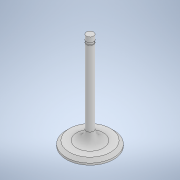
# Autodesk Inventor part: выпускной_клапан
Saved by Autodesk Inventor 2021 (Build 250183000, 183)
## iProperties
Created: 2020-12-20
Part Number: выпускной_клапан
Material: Типовые
Document SubType Name: Modeling
Designer: panda
Density: 1 g/cm^3
Appearance: По умолчанию
Author: panda
Autodesk Inventor part; units mm, degrees
ref_plane "YZ Plane" through (0, 0, 0) normal (1, 0, 0) x (0, 1, 0)
ref_plane "XZ Plane" through (0, 0, 0) normal (0, 1, 0) x (-1, 0, 0)
ref_plane "XY Plane" through (0, 0, 0) normal (0, 0, 1) x (1, 0, 0)
sketch "Эскиз1" plane through (0, 0, 0) normal (0, 0, 1) x (1, 0, 0)
  line L0 (0, 0) -> (19.5, 0)
  line L1 (19.5, 0) -> (19.5, 1.5)
  line L2 (19.5, 1.5) -> (17, 4)
  line L3 (0, 80) -> (3, 80)
  line L4 (17, 4) -> (11, 4)
  arc A0 (3, 12) -> (11, 4) centre (11, 12) ccw
  line L5 (3, 80) -> (3, 76)
  line L6 (3, 76) -> (2.5, 76)
  line L7 (2.5, 76) -> (2.5, 74)
  line L8 (2.5, 74) -> (3, 74)
  line L9 (3, 80) -> (3, 76)
  line L10 (3, 74) -> (3, 12)
  line L11 (0, 80) -> (0, 0)
  dimension "d0" = 19.5
  dimension "d1" = 1.5
  dimension "d2" = 45
  dimension "d3" = 17
  dimension "d4" = 3
  dimension "d5" = 8
  dimension "d6" = 80
  dimension "d7" = 4
  dimension "d8" = 2
  dimension "d9" = 0.5
  constraints: 24 end point, 8 perpendicular, 3 horizontal, 3 tangent, 2 point on circle, 1 centre point, 1 vertical, 1 vertical alignment
  measures "d0" distance of L0.start L0.end
  measures "d1" distance of L0.end L1.end
  measures "d2" angle of L0 L2
  measures "d3" horizontal distance of L0.start L2.end
  measures "d4" distance of L3.start L3.end
  measures "d5" radius of A0
  measures "d6" distance of L0.start L3.start
  measures "d7" distance of L3.end L5.end
  measures "d8" distance of L6.end L7.end
  measures "d9" distance of L5.end L6.end
revolve "Вращение1" add sketch "Эскиз1" angle 360 about axis through (0, 80, 0) along (0, -1, 0)
